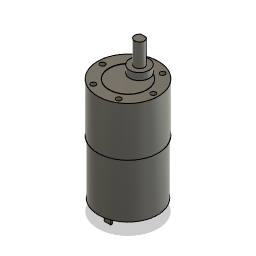
worm gear motor v6 (Autodesk Fusion 360 design; units mm, degrees)
Autodesk Fusion 360 part; units mm, degrees
sketch "Sketch1" plane through (0, 0, 0) normal (0, 1, 0) x (1, 0, 0)
  circle A0 centre (0, 0) radius 3
  circle A1 centre (0, 0) radius 6.75
  line L0 (0, 0) -> (9, 0)
  line L1 (9, 0) -> (9, -9)
  circle A2 centre (9, -9) radius 4
  circle A3 centre (9, -9) radius 1.5
  circle A4 centre (-24, -9) radius 1.5
  circle A5 centre (-24, -9) radius 4
  circle A6 centre (9, 9) radius 1.5
  circle A7 centre (9, 9) radius 4
  circle A8 centre (-24, 9) radius 1.5
  circle A9 centre (-24, 9) radius 4
  line L2 (0, 0) -> (-12, 0)
  line L3 (-12, 0) -> (-12, 6)
  line L4 (-12, 0) -> (-12, -6)
  circle A10 centre (-12, 6) radius 3.5
  circle A11 centre (-12, -6) radius 3.5
  line L5 (0, 0) -> (0, 16)
  line L6 (0, 0) -> (15.5, 0)
  line L7 (14, 16) -> (-29, 16)
  line L8 (-30.5, 14.5) -> (-30.5, -14.5)
  line L9 (-29, -16) -> (14, -16)
  line L10 (15.5, -14.5) -> (15.5, 14.5)
  arc A12 (-29, 16) -> (-30.5, 14.5) centre (-29, 14.5) ccw
  arc A13 (-30.5, -14.5) -> (-29, -16) centre (-29, -14.5) ccw
  arc A14 (14, -16) -> (15.5, -14.5) centre (14, -14.5) ccw
  arc A15 (15.5, 14.5) -> (14, 16) centre (14, 14.5) ccw
  circle A16 centre (-12, 6) radius 3
  circle A17 centre (-12, -6) radius 3
  circle A18 centre (0, 0) radius 4
  circle A19 centre (14, -14.5) radius 2.5
  circle A20 centre (13.4202, 14) radius 2.5
  arc A21 (6.1, 11.755) -> (6.9488, 12.434) centre (5, 14) ccw
  circle A22 centre (-28, 14) radius 2.5
  circle A23 centre (-21, -14) radius 2.5
  arc A24 (-30.5, -13.9986) -> (-30.5, -14.0014) centre (-28, -14) ccw
  point P0 (15.5, 16)
  point P1 (-30.5, 16)
  point P2 (15.5, -16)
  dimension "d1" = 6
  dimension "d2" = 13.5
  dimension "d3" = 9
  dimension "d4" = 9
  dimension "d5" = 8
  dimension "d6" = 3
  dimension "d9" = -33
  dimension "d10" = 18
  dimension "d11" = 12
  dimension "d12" = 6
  dimension "d13" = 6
  dimension "d14" = 7
  dimension "d15" = 7
  dimension "d16" = 16
  dimension "d17" = 15.5
  dimension "d18" = 46
  dimension "d19" = 32
  dimension "d20" = 1.5
  dimension "d32" = 6
  dimension "d33" = 6
  dimension "d34" = 8
  dimension "d46" = 5
  dimension "d47" = 5
  dimension "d52" = 5
  dimension "d53" = 5
  dimension "d54" = 5
  constraint coincident A0.centre A1.centre
  constraint horizontal L0
  constraint perpendicular L0 L1
  constraint coincident L1.end A2.centre
  constraint concentric A2 A3
  constraint parallel L0 L2
  constraint perpendicular L2 L3
  constraint perpendicular L2 L4
  constraint coincident L3.end A10.centre
  constraint coincident L4.end A11.centre
  constraint perpendicular L0 L5
  constraint perpendicular L1 L6
  constraint horizontal L7
  constraint vertical L8
  constraint horizontal L9
  constraint vertical L10
  constraint coincident P1 L7
  constraint coincident P1 L8
  constraint tangent L7 A12
  constraint tangent L8 A12
  constraint tangent L9 A13
  constraint tangent L8 A13
  constraint equal A12 A13
  constraint coincident P2 L9
  constraint coincident P2 L10
  constraint tangent L9 A14
  constraint tangent L10 A14
  constraint equal A12 A14
  constraint coincident P0 L7
  constraint coincident P0 L10
  constraint tangent L7 A15
  constraint tangent L10 A15
  constraint equal A12 A15
  constraint concentric A10 A16
  constraint concentric A11 A17
  constraint concentric A1 A18
  constraint concentric A14 A19
  constraint coincident A7 A21.start
  constraint coincident A7 A21.end
  constraint coincident L8 A24.start
  constraint coincident L8 A24.end
  measures "d1" diameter of A0
  measures "d2" diameter of A1
  measures "d3" distance of A0.centre L0.end
  measures "d4" distance of L0.end L1.end
  measures "d5" diameter of A2
  measures "d6" diameter of A3
  measures "d11" distance of A0.centre L2.end
  measures "d12" distance of L2.end L3.end
  measures "d13" distance of L2.end L4.end
  measures "d14" diameter of A10
  measures "d15" diameter of A11
  measures "d16" distance of A0.centre L5.end
  measures "d17" distance of A0.centre L6.end
  measures "d18" distance of P0 P1
  measures "d19" distance of P0 P2
  measures "d20" radius of A12
  measures "d32" diameter of A16
  measures "d33" diameter of A17
  measures "d34" diameter of A18
  measures "d46" diameter of A19
  measures "d47" diameter of A21
  measures "d52" diameter of A20
  measures "d53" diameter of A22
  measures "d54" diameter of A23
extrude "Extrude1" add sketch "Sketch1" along normal blind 2 contours A0 L0 L2 L6 A18 | A0 L0 L5 L6 A18 | A0 L2 L5 A18 | A1 L0 L5 L6 A18 | A1 L0 L2 L6 A18 | A1 L2 L5 A18 | A9 A22 | A9 A22 | A5 A23 | A5 A23 | A2 | A7 A21 | A7 A21 | A10 | A11 | A16 | A17 makes body 1 at (5.4749, 2, -0.3353) makes body 2 at (-20.005, 0.6667, -8.8006) makes body 3 at (-8.5044, 0.6667, -5.8255) makes body 4 at (12.995, 0.6667, -8.8006) makes body 5 at (-20.0199, 1.3333, 8.6017) makes body 6 at (-8.5174, 1.3333, 5.6515) makes body 7 at (12.9801, 1.3333, 8.6017)
extrude "Extrude2" add sketch "Sketch1" 7 faces at (-10.6893, 0, -5.0441) (-20.8538, 0, -8.7268) (-11.6532, 0, 7.6131) (5.4637, 0, 0.4844) (12.1462, 0, -8.7268) (12.1518, 0, 9.1987) (-20.8538, 0, 9.2732) against normal blind 21.25 contours A0 L0 L5 L6 | A0 L0 L2 L6 | A0 L2 L5 | A1 L0 A5 A9 L5 L6 L7 L8 L9 L10 A13 A19 A22 A23 A24 | A1 L0 L5 L6 L7 L10 A20 | L7 L10 A15 A20 | A9 L7 A12 A22 | L9 L10 A14 A19 | L8 A12 A22 | A5 L9 A23 | A3 | A4 | A6 | A8 picked at (13.931, 14.0895) picked at (13.9107, -14.4107) on bodies 1 2 3 4 5 6 7 bodies 3 1 2 4 5 6 7
extrude "Extrude3" cut 4 faces at (-23.5429, 0, -8.4269) (-23.5429, 0, 9.5731) (8.2215, 0, -8.7183) (8.1569, 0, 9.1474) along direction (0, -1, 0) blind 6 on bodies 3 bodies 3
extrude "Extrude4" add 1 faces at (1.3956, 0, 0.2284) along direction (0, 1, 0) blind 16 on bodies 3 bodies 3
sketch "Sketch2" plane through (0, 16, 0) normal (0, 1, 0) x (-1, 0, 0)
  circle A0 centre (0, 0) radius 3
  line L0 (0, 0) -> (0, -1.5)
  line L1 (2.5981, -1.5) -> (-2.5981, -1.5)
  dimension "d29" = 1.5
  constraint coincident A0.centre L0.start
  constraint vertical L0
  constraint coincident A0 L1.start
  constraint coincident A0 L1.end
  constraint perpendicular L0 L1
  measures "d29" distance of A0.centre L0.end
extrude "Extrude5" cut sketch "Sketch2" against normal blind 10.5 contours A0 L1 picked at (-0.149, -2.4888) bodies 3
extrude "Extrude6" add sketch "Sketch1" against normal blind 23 contours A0 L0 L5 L6 | A0 L0 L2 L6 A18 | A0 L0 L2 L6 | A0 L0 L5 L6 A18 | A0 L2 L5 | A0 L2 L5 A18 | A16 | A17 bodies 3
sketch "Sketch3" plane through (-30.5, 0, 0) normal (-1, 0, 0) x (0, 0, 1)
  line L0 (14.5, 0) -> (-14.5, 0)
  line L1 (-14.5, 0) -> (-14.5, -21.25)
  line L2 (-14.5, -21.25) -> (14.5, -21.25)
  line L3 (14.5, -21.25) -> (14.5, 0)
  line L4 (-14.5, -10.625) -> (-15.5, -10.625)
  line L5 (-15.5, -10.625) -> (-3.5, -10.625)
  line L6 (-2, -21.25) -> (-2, -12.75)
  circle A0 centre (-2, -12.75) radius 12
  dimension "d37" = 1
  dimension "d38" = 12
  dimension "d39" = 8.5
  dimension "d40" = 24
  constraint midpoint L1 L4.start
  constraint perpendicular L1 L4
  constraint perpendicular L1 L5
  constraint coincident L2 L6.start
  constraint perpendicular L2 L6
  constraint coincident L6.end A0.centre
  measures "d37" distance of L4.start L4.end
  measures "d38" distance of L4.end L5.end
  measures "d39" distance of L6.start L6.end
  measures "d40" diameter of A0
extrude "Extrude7" add sketch "Sketch3" along normal blind 30.5 contours L2 A0 | L2 A0 bodies 3
sketch "Sketch4" plane through (-61, 0, 0) normal (-1, 0, 0) x (0, 0, 1)
  circle A0 centre (-2, -12.75) radius 12
  circle A1 centre (-2, -12.75) radius 3.175
  dimension "d43" = 6.35
  constraint concentric A0 A1
  measures "d43" diameter of A1
extrude "Extrude8" add sketch "Sketch4" along normal blind 1 contours A1 bodies 3
extrude "Extrude9" add sketch "Sketch1" along normal blind 2 contours L7 L10 A15 A20 | A9 L7 A12 A22 | L9 L10 A14 A19 | L8 A12 A22 | A9 A22 | A5 L9 A23 | A7 A21 picked at (13.931, 14.0895) picked at (13.9107, -14.4107) picked at (-26.7076, 11.9003) picked at (6.7648, 12.2782) bodies 3
sketch "Sketch5" plane through (0, 0, 0) normal (0, 1, 0) x (1, 0, 0)
  circle A0 centre (0, 0) radius 18.5
  circle A1 centre (0, 0) radius 18
  dimension "d55" = 37
  dimension "d56" = 36
  constraint coincident A0.centre A1.centre
  measures "d55" diameter of A0
  measures "d56" diameter of A1
extrude "Extrude10" add sketch "Sketch5" against normal blind 33 separate body contours A1 makes body 8
extrude "Extrude11" add sketch "Sketch5" along normal blind 30 contours A0 | A1 bodies 8
sketch "Sketch6" plane through (0, 30, 0) normal (0, 1, 0) x (-1, 0, 0)
  circle A0 centre (0, 0) radius 18.5
  line L0 (0, 0) -> (-15.5, 0) construction
  circle A1 centre (-15.5, 0) radius 1.5
  circle A2 centre (-7.75, -13.4234) radius 1.5
  circle A3 centre (7.75, -13.4234) radius 1.5
  circle A4 centre (15.5, 0) radius 1.5
  circle A5 centre (7.75, 13.4234) radius 1.5
  circle A6 centre (-7.75, 13.4234) radius 1.5
  line L1 (0, 0) -> (0, -7) construction
  circle A7 centre (0, -7) radius 6
  circle A8 centre (0, -7) radius 3
  circle A9 centre (0, 0) radius 11.5
  dimension "d61" = 15.5
  dimension "d62" = 3
  dimension "d64" = 360
  dimension "d65" = 7
  dimension "d66" = 12
  dimension "d67" = 6
  dimension "d85" = 23
  constraint coincident A0.centre L0.start
  constraint horizontal L0
  constraint coincident L0.end A1.centre
  constraint perpendicular L0 L1
  constraint coincident L1.end A7.centre
  constraint concentric A7 A8
  measures "d61" distance of A0.centre L0.end
  measures "d62" diameter of A1
  measures "d65" distance of A0.centre L1.end
  measures "d66" diameter of A7
  measures "d67" diameter of A8
  measures "d85" diameter of A9
extrude "Extrude17" cut sketch "Sketch6" against normal blind 0.25 contours A7 A9 picked at (0.3496, 7.3044) bodies 8
extrude "Extrude12" cut sketch "Sketch6" against normal blind 5 contours A1 | A2 | A3 | A4 | A5 | A6 bodies 8
extrude "Extrude13" add sketch "Sketch6" along normal blind 18 contours A8 bodies 8
extrude "Extrude14" add sketch "Sketch6" along normal blind 4 contours A7 A9 | A7 A9 picked at (-3.6029, -10.0201) picked at (1.0133, -11.9075) bodies 8
sketch "Sketch7" plane through (0, -33, 0) normal (0, -1, 0) x (1, 0, 0)
  circle A0 centre (0, 0) radius 18
  circle A1 centre (0, 0) radius 5
  line L0 (0, 0) -> (0, -12) construction
  line L1 (-2, -11.6) -> (2, -11.6)
  line L2 (2, -11.6) -> (2, -12.4)
  line L3 (2, -12.4) -> (-2, -12.4)
  line L4 (-2, -12.4) -> (-2, -11.6)
  line L5 (-2, -11.6) -> (2, -12.4) construction
  line L6 (2, -11.6) -> (-2, -12.4) construction
  line L7 (0, 0) -> (0, 12) construction
  line L8 (-2, 12.5) -> (2, 12.5)
  line L9 (2, 12.5) -> (2, 11.5)
  line L10 (2, 11.5) -> (-2, 11.5)
  line L11 (-2, 11.5) -> (-2, 12.5)
  line L12 (-2, 12.5) -> (2, 11.5) construction
  line L13 (2, 12.5) -> (-2, 11.5) construction
  point P0 (0, -12)
  point P1 (0, 12)
  dimension "d74" = 10
  dimension "d78" = 12
  dimension "d79" = 4
  dimension "d80" = 12
  dimension "d81" = 4
  dimension "d82" = 1
  constraint concentric A0 A1
  constraint coincident A0.centre A1.centre
  constraint vertical L0
  constraint horizontal L1
  constraint perpendicular L1 L2
  constraint parallel L1 L3
  constraint parallel L2 L4
  constraint coincident L5 P0
  constraint coincident L6 P0
  constraint coincident P0 L0.end
  constraint parallel L0 L7
  constraint horizontal L8
  constraint perpendicular L8 L9
  constraint parallel L8 L10
  constraint parallel L9 L11
  constraint coincident L12 P1
  constraint coincident L13 P1
  constraint coincident P1 L7.end
  measures "d74" diameter of A1
  measures "d78" distance of A0.centre P0
  measures "d79" distance of L2.end L3.end
  measures "d80" distance of A0.centre P1
  measures "d81" distance of L9.end L10.end
  measures "d82" distance of L8.end L9.end
extrude "Extrude16" add sketch "Sketch7" along normal blind 7 contours L1 L2 L3 L4 | L8 L9 L10 L11 bodies 8
extrude "Extrude15" add sketch "Sketch7" along normal blind 4 contours A1 bodies 8
chamfer "Chamfer1" distance 2 angle 45 1 edges at (-4.6616, -37, -1.8081) on bodies 8
copy_body "Body->Comp1" bodies 8 removing the originals makes body 9 in component "spur gear motor"
sketch "Sketch8" plane through (0, 48, 0) normal (0, 1, 0) x (-1, 0, 0)
  circle A0 centre (0, -7) radius 3
  line L0 (0, -4) -> (0, -9.5) construction
  line L1 (1.6583, -9.5) -> (-1.6583, -9.5)
  dimension "d88" = 5.5
  constraint coincident A0 L0.start
  constraint vertical L0
  constraint coincident A0 L1.start
  constraint coincident A0 L1.end
  constraint perpendicular L0 L1
  measures "d88" distance of L0.start L0.end
extrude "Extrude1'" cut sketch "Sketch8" against normal blind 13.5 contours A0 L1 picked at (0.4253, -9.5717) bodies 9 in component "spur gear motor"
component "spur gear motor" placed x (1, 0, 0) y (0, 1, 0) z (0, 0, 1) at (0, 0, 0)
hidden bodies 3
equation "d17 = 9 mm + ( ( 46 - 33 ) / 2 ) * 1 mm"
equation "d29 = 6 mm - 4.5 mm"
equation "d38 = ( 24 / 2 ) * 1 mm"
equation "d39 = 12 mm - 3.5 mm"
equation "d43 = ( 25.4 / 4 ) * 1 mm"
equation "d61 = ( 31 / 2 ) * 1 mm"
